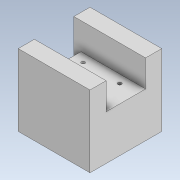
# Autodesk Inventor part: IMU_Calibration_Cube
Saved by Autodesk Inventor 2020 (Build 240168000, 168)
## iProperties
Created: 2021-05-08
Part Number: IMU_Calibration_Cube
Material: Generic
Document SubType Name: Modeling
Designer: DELL
Density: 1 g/cm^3
Appearance: Default
Author: DELL
Autodesk Inventor part; units mm, degrees
ref_plane "YZ Plane" through (0, 0, 0) normal (1, 0, 0) x (0, 1, 0)
ref_plane "XZ Plane" through (0, 0, 0) normal (0, 1, 0) x (-1, 0, 0)
ref_plane "XY Plane" through (0, 0, 0) normal (0, 0, 1) x (1, 0, 0)
sketch "Sketch1" plane through (0, 0, 0) normal (0, 1, 0) x (-1, 0, 0)
  line L0 (-20, -20) -> (20, -20)
  line L1 (20, -20) -> (20, 20)
  line L2 (20, 20) -> (-20, 20)
  line L3 (-20, 20) -> (-20, -20)
  line L4 (-20, -20) -> (20, 20) construction
  line L5 (20, -20) -> (-20, 20) construction
  point P0 (0, 0)
  dimension "d0" = 40
  constraints: 12 end point, 2 midpoint, 2 parallel, 2 perpendicular, 1 horizontal
  measures "d0" distance of L0.end L1.end
extrude "Extrusion1" add sketch "Sketch1" along normal mid plane 40
sketch "Sketch2" plane through (0, 20, 0) normal (0, 1, 0) x (1, 0, 0)
  line L0 (-20, 20) -> (-20, -20) projected
  line L1 (20, -11) -> (-20, -11)
  line L2 (-20, -11) -> (-20, 11)
  line L3 (-20, 11) -> (20, 11)
  line L4 (20, 11) -> (20, -11)
  line L5 (20, -11) -> (-20, 11) construction
  line L6 (-20, -11) -> (20, 11) construction
  line L7 (-24, -11) -> (-16, -11)
  line L8 (-16, -11) -> (-16, 11)
  line L9 (-16, 11) -> (-24, 11)
  line L10 (-24, 11) -> (-24, -11)
  line L11 (-24, -11) -> (-16, 11) construction
  line L12 (-16, -11) -> (-24, 11) construction
  line L13 (-10.16, 6.35) -> (10.16, 6.35) construction
  line L14 (10.16, 6.35) -> (10.16, -6.35) construction
  line L15 (10.16, -6.35) -> (-10.16, -6.35) construction
  line L16 (-10.16, -6.35) -> (-10.16, 6.35) construction
  line L17 (-10.16, 6.35) -> (10.16, -6.35) construction
  line L18 (10.16, 6.35) -> (-10.16, -6.35) construction
  circle A0 centre (10.16, -6.35) radius 1
  circle A1 centre (-10.16, -6.35) radius 1
  circle A2 centre (-10.16, 6.35) radius 1
  circle A3 centre (10.16, 6.35) radius 1
  point P0 (0, 0)
  point P1 (-20, -11)
  point P2 (-20, 0)
  point P3 (-20, -11)
  point P4 (-16, -11)
  dimension "d3" = 22
  dimension "d6" = 8
  dimension "d9" = 12.7
  dimension "d10" = 20.32
  dimension "d11" = 2
  constraints: 36 end point, 7 midpoint, 6 parallel, 4 centre point, 4 coincident, 3 equal radius, 3 horizontal, 3 perpendicular, 2 point on line
  measures "d3" distance between parallel lines of L1 L3
  measures "d6" distance between parallel lines of L10 L8
  measures "d9" distance of L13.end L14.end
  measures "d10" distance of L14.end L15.end
  measures "d11" diameter of A0
extrude "Extrusion2" cut sketch "Sketch2" against normal blind 15 contours L3 L8 L1 L0 | L3 L4 L1 L8 | A0 | A1 | A2 | A3
extrude "Extrusion3" cut sketch "Sketch2" against normal through all contours L3 L8 L1 L0 | L0 L7 L10 L9
extrude "Extrusion4" cut sketch "Sketch2" against normal through all contours A0 | A1 | A2 | A3
body "Solid1"
